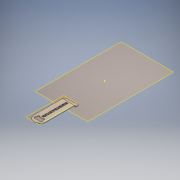
# Autodesk Inventor part: Rost_Heber
Saved by Autodesk Inventor 2018 (Build 220112000, 112)
## iProperties
Created: 2017-10-08
Part Number: Rost_Heber
Material: Generisch
Document SubType Name: Blech
Designer: Jan
Density: 1 g/cm^3
Sheet Metal Rule: Standard_mm
Appearance: Vorgabe
Flat Pattern Width: 4 cm
Flat Pattern Length: 13.3098 cm
Flat Pattern Area: 53.2391 cm^2
Sheet Metal Width: 40,000 mm
Sheet Metal Length: 133,098 mm
Sheet Metal Area: 5323,911 mm^2
Author: Jan
Autodesk Inventor part; units mm, degrees
ref_plane "YZ Plane" through (0, 0, 0) normal (1, 0, 0) x (0, 1, 0)
ref_plane "XZ Plane" through (0, 0, 0) normal (0, 1, 0) x (-1, 0, 0)
ref_plane "XY Plane" through (0, 0, 0) normal (0, 0, 1) x (1, 0, 0)
ref_plane "Arbeitsebene1" through (0, 0, 0) normal (0, 0, 1) x (1, 0, 0)
sketch "Skizze1" plane through (0, 0, 0) normal (0, 0, 1) x (1, 0, 0)
  arc A0 (31.5, -113.5) -> (26.5, -108.5) centre (26.5, -113.5) ccw
  line L0 (26.5, -108.5) -> (-26.5, -108.5)
  arc A1 (-26.5, -108.5) -> (-31.5, -113.5) centre (-26.5, -113.5) ccw
  line L1 (-31.5, -113.5) -> (-31.5, -124.5)
  line L2 (-31.5, -124.5) -> (-71, -124.5)
  arc A2 (-73, -122.5) -> (-71, -124.5) centre (-71, -122.5) ccw
  line L3 (-73, -122.5) -> (-73, 122.5)
  arc A3 (-71, 124.5) -> (-73, 122.5) centre (-71, 122.5) ccw
  line L4 (-71, 124.5) -> (71, 124.5)
  arc A4 (73, 122.5) -> (71, 124.5) centre (71, 122.5) ccw
  line L5 (73, 122.5) -> (73, -122.5)
  arc A5 (71, -124.5) -> (73, -122.5) centre (71, -122.5) ccw
  line L6 (71, -124.5) -> (31.5, -124.5)
  line L7 (31.5, -124.5) -> (31.5, -113.5)
  line L8 (-22.5, -122.5) -> (-22.5, -117.5)
  line L9 (-22.5, -117.5) -> (22.5, -117.5)
  line L10 (22.5, -117.5) -> (22.5, -122.5)
  line L11 (22.5, -122.5) -> (-22.5, -122.5)
  arc A6 (-81, -122.5) -> (-71, -132.5) centre (-71, -122.5) ccw
  line L12 (71, -132.5) -> (-71, -132.5)
  arc A7 (71, -132.5) -> (81, -122.5) centre (71, -122.5) ccw
  line L13 (81, 122.5) -> (81, -122.5)
  arc A8 (81, 122.5) -> (71, 132.5) centre (71, 122.5) ccw
  line L14 (-71, 132.5) -> (71, 132.5)
  arc A9 (-71, 132.5) -> (-81, 122.5) centre (-71, 122.5) ccw
  line L15 (-81, -122.5) -> (-81, 122.5)
  line L16 (-20, -118.5) -> (20, -118.5)
  line L17 (20, -118.5) -> (20, -218.5)
  line L18 (0, -238.5) -> (0, -238.5)
  line L19 (-20, -218.5) -> (-20, -118.5)
  line L20 (-116.2995, 0) -> (116.2995, 0)
  line L21 (0, -314.1009) -> (0, 209.3497)
  arc A10 (-20, -218.5) -> (0, -238.5) centre (0, -218.5) ccw
  arc A11 (0, -238.5) -> (20, -218.5) centre (0, -218.5) ccw
  point P0 (0, 0)
  dimension "HeberBreite" = 40
  dimension "d3" = 1
  dimension "HeberLänge" = 120
  dimension "d5" = 20
  measures "HeberBreite" distance of L16.start L16.end
  measures "d3" distance between parallel lines of L9 L16
  measures "HeberLänge" distance between parallel lines of L18 L16
  measures "d5" radius of A10
extrude "Grobblech1" add sketch "Skizze1" along normal blind 2 contours L21 L11 L19 L16 | L16 L17 L11 L21 | L21 L12 L19 L11 | L11 L17 L12 L21 | L21 A10 L19 L12 | L12 L17 A11 L21
sketch "Skizze2" plane through (20, -120.5, 2) normal (0, 1, 0) x (-1, 0, 0)
  line L0 (40, 0) -> (0, 0)
  line L1 (0, 0) -> (0, -8.05)
  line L2 (0, -8.05) -> (40, -8.05)
  line L3 (40, -8.05) -> (40, 0)
  constraints: 6 end point, 1 horizontal, 1 perpendicular, 1 vertical
edge flange "Lasche1" height 8.05 angle 90 thickness 2 bend radius 2 thickness toward (0, 1, 0) relief straight relief width 2 relief depth 1 edges at (0, -118.5, 0) wall of the first edge with corners at (-20, -120.5, 2) (20, -120.5, 2) (20, -120.5, -6.05) (-20, -120.5, -6.05)
bend "Biegung1"
corner "Ecke1"
sketch "Skizze3" plane through (-20, -120.5, -4.05) normal (0, 0, -1) x (-1, 0, 0)
  line L0 (-40, 0) -> (0, 0)
  line L1 (0, 0) -> (0, 12)
  line L2 (0, 12) -> (-40, 12)
  line L3 (-40, 12) -> (-40, 0)
  constraints: 6 end point, 1 horizontal, 1 perpendicular, 1 vertical
edge flange "Lasche2" height 12 angle 90 thickness 2 bend radius 2 thickness toward (0, 0, -1) relief straight relief width 2 relief depth 1 edges at (0, -118.5, -6.05) wall of the first edge with corners at (20, -120.5, -4.05) (-20, -120.5, -4.05) (-20, -108.5, -4.05) (20, -108.5, -4.05)
bend "Biegung2"
corner "Ecke2"
sketch "Skizze5" plane through (0, 0, 2) normal (0, 0, 1) x (1, 0, 0)
  line L0 (6.947, -214.5463) -> (6.947, -212.4824)
  arc A0 (10.3384, -213.2197) -> (6.947, -212.4824) centre (8.3903, -214.0121) ccw
  line L1 (10.3384, -213.2197) -> (13.6109, -223.4321)
  arc A1 (4.1757, -228.0984) -> (13.6109, -223.4321) centre (7.6304, -223.2116) ccw
  line L2 (20, -122.5) -> (-20, -122.5) projected
  line L3 (-20, -218.5) -> (-20, -122.5) projected
  arc A2 (-20, -218.5) -> (20, -218.5) centre (0, -218.5) ccw projected
  line L4 (20, -122.5) -> (20, -218.5) projected
  line L5 (6.947, -214.5463) -> (-0.053, -214.5463)
  line L6 (4.1757, -228.0984) -> (-0.053, -228.0984)
  arc A3 (-7.053, -212.4824) -> (-10.3568, -213.0318) centre (-8.4962, -214.0121) ccw
  line L7 (-10.3568, -213.0318) -> (-13.7136, -223.5071)
  arc A4 (-13.7136, -223.5071) -> (-4.2816, -228.0984) centre (-7.7363, -223.2116) ccw
  line L8 (-7.053, -214.5463) -> (-0.053, -214.5463)
  line L9 (-4.2816, -228.0984) -> (-0.053, -228.0984)
  line L10 (-7.053, -212.4824) -> (-7.053, -214.5463)
  line L11 (0, -312.7) -> (0, 206.7)
  constraints: 19 end point, 8 point on circle, 4 centre point, 3 parallel, 2 equal radius, 1 point on line, 1 vertical, 2 other
extrude "Ausklinkung1" cut sketch "Skizze5" against normal blind 2 contours L0 A0 L1 A1 L6 L11 L5 | L11 L6 L9 A4 L7 A3 L10 L8 L5
sketch "Skizze7" plane through (0, 0, 2) normal (0, 0, 1) x (1, 0, 0)
  point P0 (0, 0)
ref_plane "Arbeitsebene2" through (0, 0, 7) normal (0, 0, 1) x (1, 0, 0)
sketch "Skizze8" plane through (0, 0, 7) normal (0, 0, 1) x (1, 0, 0)
  line L0 (3.8058, -125.538) -> (3.8058, -288.8575) construction
  line L1 (3.8058, -288.8575) -> (-4.5136, -288.8575) construction
  line L2 (-4.5136, -288.8575) -> (-4.5136, -125.538) construction
  line L3 (-4.5136, -125.538) -> (3.8058, -125.538) construction
  line L4 (3.6661, -129.3965) -> (-3.3339, -129.3965)
  line L5 (-3.3339, -129.3965) -> (-3.3339, -126.6622)
  line L6 (-3.3339, -126.6622) -> (-3.3339, -126.5042)
  spline S0 degree 2 poles (-3.3339, -126.5042) (-3.3339, -126.2794) (-3.1942, -126.0424) (-3.0666, -126.0424) knots 0 0 0 1 2 2 2
  spline S1 degree 2 poles (-3.0666, -126.0424) (-2.86, -126.0424) (-2.7931, -126.2854) knots 0 0 0 1 1 1
  spline S2 degree 2 poles (-2.7931, -126.2854) (-2.7324, -126.492) (-2.7081, -126.5589) (-2.6595, -126.5953) knots 0 0 0 1 2 2 2
  spline S3 degree 2 poles (-2.6595, -126.5953) (-2.5805, -126.6682) (-2.3982, -126.6682) knots 0 0 0 1 1 1
  line L7 (-2.3982, -126.6682) -> (2.7303, -126.6682)
  spline S4 degree 2 poles (2.7303, -126.6682) (2.9126, -126.6682) (2.9916, -126.5953) knots 0 0 0 1 1 1
  spline S5 degree 2 poles (2.9916, -126.5953) (3.0402, -126.5589) (3.0645, -126.492) (3.1192, -126.2854) knots 0 0 0 1 2 2 2
  spline S6 degree 2 poles (3.1192, -126.2854) (3.186, -126.0424) (3.3987, -126.0424) knots 0 0 0 1 1 1
  spline S7 degree 2 poles (3.3987, -126.0424) (3.5263, -126.0424) (3.6661, -126.2794) (3.6661, -126.5042) knots 0 0 0 1 2 2 2
  line L8 (3.6661, -126.5042) -> (3.6661, -126.6622)
  line L9 (3.6661, -126.6622) -> (3.6661, -129.3965)
  line L10 (-3.3339, -129.9556) -> (-2.781, -129.9556)
  spline S8 degree 2 poles (-2.781, -129.9556) (-2.7324, -130.3566) (-2.544, -130.8792) (-2.3556, -131.1405) knots 0 0 0 1 2 2 2
  spline S9 degree 2 poles (-2.3556, -131.1405) (-2.1673, -131.4078) (-1.7602, -131.7177) (-1.4259, -131.8636) knots 0 0 0 1 2 2 2
  spline S10 degree 2 poles (-1.4259, -131.8636) (-1.2619, -131.9304) (-1.1464, -132.0762) (-1.1464, -132.2038) knots 0 0 0 1 2 2 2
  spline S11 degree 2 poles (-1.1464, -132.2038) (-1.1464, -132.3801) (-1.3166, -132.5137) (-1.5232, -132.5137) knots 0 0 0 1 2 2 2
  line L11 (-1.5232, -132.5137) -> (-3.3339, -132.5137)
  line L12 (-3.3339, -132.5137) -> (-3.3339, -129.9556)
  line L13 (3.6661, -129.9495) -> (3.6661, -132.4287)
  line L14 (3.6661, -132.4287) -> (1.8492, -132.4287)
  spline S12 degree 2 poles (1.8492, -132.4287) (1.6912, -132.4287) (1.5515, -132.2828) (1.5515, -132.1188) knots 0 0 0 1 2 2 2
  spline S13 degree 2 poles (1.5515, -132.1188) (1.5515, -131.9851) (1.6426, -131.8636) (1.7885, -131.8089) knots 0 0 0 1 2 2 2
  spline S14 degree 2 poles (1.7885, -131.8089) (2.3779, -131.5719) (3.0037, -130.6665) (3.0645, -129.9495) knots 0 0 0 1 2 2 2
  line L15 (3.0645, -129.9495) -> (3.6661, -129.9495)
  line L16 (-0.0709, -129.9191) -> (0.5246, -129.9191)
  spline S15 degree 2 poles (0.5246, -129.9191) (0.6704, -130.2776) (1.0107, -130.6179) (1.2902, -130.703) knots 0 0 0 1 2 2 2
  spline S16 degree 2 poles (1.2902, -130.703) (1.4846, -130.7516) (1.6366, -130.9096) (1.6366, -131.0554) knots 0 0 0 1 2 2 2
  spline S17 degree 2 poles (1.6366, -131.0554) (1.6366, -131.2559) (1.5089, -131.3288) knots 0 0 0 1 1 1
  spline S18 degree 2 poles (1.5089, -131.3288) (1.4421, -131.3714) (1.2051, -131.3714) knots 0 0 0 1 1 1
  line L17 (1.2051, -131.3714) -> (-0.7515, -131.3714)
  spline S19 degree 2 poles (-0.7515, -131.3714) (-0.9945, -131.3714) (-1.1768, -131.2438) (-1.1768, -131.0676) knots 0 0 0 1 2 2 2
  spline S20 degree 2 poles (-1.1768, -131.0676) (-1.1768, -130.9278) (-1.031, -130.7698) (-0.8608, -130.7212) knots 0 0 0 1 2 2 2
  spline S21 degree 2 poles (-0.8608, -130.7212) (-0.5084, -130.6118) (-0.1317, -130.229) (-0.0709, -129.9191) knots 0 0 0 1 2 2 2
  line L18 (-3.3339, -136.7976) -> (-3.3339, -134.0571)
  line L19 (-3.3339, -134.0571) -> (-3.3339, -133.8992)
  spline S22 degree 2 poles (-3.3339, -133.8992) (-3.3339, -133.6743) (-3.1942, -133.4373) (-3.0666, -133.4373) knots 0 0 0 1 2 2 2
  spline S23 degree 2 poles (-3.0666, -133.4373) (-2.86, -133.4373) (-2.7931, -133.6804) knots 0 0 0 1 1 1
  spline S24 degree 2 poles (-2.7931, -133.6804) (-2.7324, -133.887) (-2.7081, -133.9538) (-2.6595, -133.9903) knots 0 0 0 1 2 2 2
  spline S25 degree 2 poles (-2.6595, -133.9903) (-2.5805, -134.0632) (-2.3982, -134.0632) knots 0 0 0 1 1 1
  line L20 (-2.3982, -134.0632) -> (2.7303, -134.0632)
  spline S26 degree 2 poles (2.7303, -134.0632) (2.9126, -134.0632) (2.9916, -133.9903) knots 0 0 0 1 1 1
  spline S27 degree 2 poles (2.9916, -133.9903) (3.0402, -133.9538) (3.0645, -133.887) (3.1192, -133.6804) knots 0 0 0 1 2 2 2
  spline S28 degree 2 poles (3.1192, -133.6804) (3.186, -133.4373) (3.3987, -133.4373) knots 0 0 0 1 1 1
  spline S29 degree 2 poles (3.3987, -133.4373) (3.5263, -133.4373) (3.6661, -133.6743) (3.6661, -133.8992) knots 0 0 0 1 2 2 2
  line L21 (3.6661, -133.8992) -> (3.6661, -134.0571)
  line L22 (3.6661, -134.0571) -> (3.6661, -136.7976)
  line L23 (3.6661, -136.7976) -> (3.6661, -136.9556)
  spline S30 degree 2 poles (3.6661, -136.9556) (3.6661, -137.1804) (3.5263, -137.4174) (3.3987, -137.4174) knots 0 0 0 1 2 2 2
  spline S31 degree 2 poles (3.3987, -137.4174) (3.186, -137.4174) (3.1192, -137.1743) knots 0 0 0 1 1 1
  spline S32 degree 2 poles (3.1192, -137.1743) (3.0645, -136.9677) (3.0402, -136.9009) (2.9916, -136.8644) knots 0 0 0 1 2 2 2
  spline S33 degree 2 poles (2.9916, -136.8644) (2.9126, -136.7915) (2.7303, -136.7915) knots 0 0 0 1 1 1
  line L24 (2.7303, -136.7915) -> (-2.3982, -136.7915)
  spline S34 degree 2 poles (-2.3982, -136.7915) (-2.5805, -136.7915) (-2.6595, -136.8644) knots 0 0 0 1 1 1
  spline S35 degree 2 poles (-2.6595, -136.8644) (-2.7081, -136.9009) (-2.7324, -136.9677) (-2.7931, -137.1743) knots 0 0 0 1 2 2 2
  spline S36 degree 2 poles (-2.7931, -137.1743) (-2.86, -137.4174) (-3.0666, -137.4174) knots 0 0 0 1 1 1
  spline S37 degree 2 poles (-3.0666, -137.4174) (-3.1942, -137.4174) (-3.3339, -137.1804) (-3.3339, -136.9556) knots 0 0 0 1 2 2 2
  line L25 (-3.3339, -136.9556) -> (-3.3339, -136.7976)
  line L26 (3.8058, -141.2698) -> (3.2164, -141.2698)
  spline S38 degree 2 poles (3.2164, -141.2698) (3.1253, -140.887) (2.7607, -140.486) (2.4994, -140.486) knots 0 0 0 1 2 2 2
  spline S39 degree 2 poles (2.4994, -140.486) (2.2381, -140.486) (1.8553, -140.8202) (1.6791, -141.1908) knots 0 0 0 1 2 2 2
  spline S40 degree 2 poles (1.6791, -141.1908) (1.5636, -141.4521) (1.2294, -142.3636) knots 0 0 0 1 1 1
  spline S41 degree 2 poles (1.2294, -142.3636) (1.0289, -142.9165) (0.7069, -143.5242) (0.4638, -143.7976) knots 0 0 0 1 2 2 2
  spline S42 degree 2 poles (0.4638, -143.7976) (-0.1681, -144.5207) (-1.0492, -144.5207) knots 0 0 0 1 1 1
  spline S43 degree 2 poles (-1.0492, -144.5207) (-1.7055, -144.5207) (-2.8053, -143.7307) (-3.1213, -143.0441) knots 0 0 0 1 2 2 2
  spline S44 degree 2 poles (-3.1213, -143.0441) (-3.2853, -142.6735) (-3.4737, -141.7985) (-3.4737, -141.4156) knots 0 0 0 1 2 2 2
  line L27 (-3.4737, -141.4156) -> (-2.8904, -141.4156)
  spline S45 degree 2 poles (-2.8904, -141.4156) (-2.781, -141.9504) (-2.3982, -142.4243) (-2.07, -142.4243) knots 0 0 0 1 2 2 2
  spline S46 degree 2 poles (-2.07, -142.4243) (-1.7237, -142.4243) (-1.4624, -142.0537) knots 0 0 0 1 1 1
  spline S47 degree 2 poles (-1.4624, -142.0537) (-1.2923, -141.8106) (-1.0431, -141.1179) knots 0 0 0 1 1 1
  spline S48 degree 2 poles (-1.0431, -141.1179) (-0.7636, -140.3644) (-0.5266, -139.8054) (-0.3687, -139.5441) knots 0 0 0 1 2 2 2
  spline S49 degree 2 poles (-0.3687, -139.5441) (0.318, -138.3896) (1.4603, -138.3896) knots 0 0 0 1 1 1
  spline S50 degree 2 poles (1.4603, -138.3896) (2.0437, -138.3896) (3.0341, -138.9669) (3.3379, -139.4834) knots 0 0 0 1 2 2 2
  spline S51 degree 2 poles (3.3379, -139.4834) (3.7572, -140.2064) (3.8058, -141.2698) knots 0 0 0 1 1 1
  line L28 (-2.8904, -140.9478) -> (-3.4737, -140.9478)
  spline S52 degree 2 poles (-3.4737, -140.9478) (-3.4737, -140.4434) (-3.2367, -139.8358) knots 0 0 0 1 1 1
  spline S53 degree 2 poles (-3.2367, -139.8358) (-3.1456, -139.6049) (-3.097, -139.4347) (-3.097, -139.3557) knots 0 0 0 1 2 2 2
  spline S54 degree 2 poles (-3.097, -139.3557) (-3.097, -139.2342) (-3.1638, -139.1066) (-3.2975, -138.9729) knots 0 0 0 1 2 2 2
  spline S55 degree 2 poles (-3.2975, -138.9729) (-3.4069, -138.8636) (-3.4069, -138.736) knots 0 0 0 1 1 1
  spline S56 degree 2 poles (-3.4069, -138.736) (-3.4069, -138.3896) (-2.9633, -138.3896) knots 0 0 0 1 1 1
  line L29 (-2.9633, -138.3896) -> (-1.0978, -138.3896)
  spline S57 degree 2 poles (-1.0978, -138.3896) (-0.9581, -138.3896) (-0.7575, -138.584) (-0.7515, -138.736) knots 0 0 0 1 2 2 2
  spline S58 degree 2 poles (-0.7515, -138.736) (-0.7454, -138.8696) (-0.8852, -139.0215) (-1.0614, -139.0762) knots 0 0 0 1 2 2 2
  spline S59 degree 2 poles (-1.0614, -139.0762) (-1.4989, -139.2221) (-2.2706, -139.7568) (-2.5319, -140.1092) knots 0 0 0 1 2 2 2
  spline S60 degree 2 poles (-2.5319, -140.1092) (-2.8114, -140.4738) (-2.8904, -140.9478) knots 0 0 0 1 1 1
  line L30 (3.2164, -141.7559) -> (3.7815, -141.7559)
  spline S61 degree 2 poles (3.7815, -141.7559) (3.7572, -142.1266) (3.6357, -142.6674) (3.4595, -143.1656) knots 0 0 0 1 2 2 2
  spline S62 degree 2 poles (3.4595, -143.1656) (3.4169, -143.2872) (3.4169, -143.3662) knots 0 0 0 1 1 1
  spline S63 degree 2 poles (3.4169, -143.3662) (3.4169, -143.4816) (3.4838, -143.5424) knots 0 0 0 1 1 1
  line L31 (3.4838, -143.5424) -> (3.6357, -143.6761)
  spline S64 degree 2 poles (3.6357, -143.6761) (3.7511, -143.7733) (3.7511, -143.913) knots 0 0 0 1 1 1
  spline S65 degree 2 poles (3.7511, -143.913) (3.7511, -144.0832) (3.5506, -144.2351) (3.3379, -144.2351) knots 0 0 0 1 2 2 2
  line L32 (3.3379, -144.2351) -> (1.6426, -144.2351)
  spline S66 degree 2 poles (1.6426, -144.2351) (1.4907, -144.2351) (1.3023, -144.0346) (1.3023, -143.8705) knots 0 0 0 1 2 2 2
  spline S67 degree 2 poles (1.3023, -143.8705) (1.3023, -143.749) (1.3692, -143.6457) knots 0 0 0 1 1 1
  spline S68 degree 2 poles (1.3692, -143.6457) (1.4117, -143.591) (1.5272, -143.5242) (1.6669, -143.4938) knots 0 0 0 1 2 2 2
  spline S69 degree 2 poles (1.6669, -143.4938) (1.9221, -143.4209) (2.4508, -143.0927) (2.6635, -142.8679) knots 0 0 0 1 2 2 2
  spline S70 degree 2 poles (2.6635, -142.8679) (3.0827, -142.4243) (3.2164, -141.7559) knots 0 0 0 1 1 1
  line L33 (3.6661, -148.841) -> (-3.3339, -148.841)
  line L34 (-3.3339, -148.841) -> (-3.3339, -146.1066)
  line L35 (-3.3339, -146.1066) -> (-3.3339, -145.9486)
  spline S71 degree 2 poles (-3.3339, -145.9486) (-3.3339, -145.7238) (-3.1942, -145.4868) (-3.0666, -145.4868) knots 0 0 0 1 2 2 2
  spline S72 degree 2 poles (-3.0666, -145.4868) (-2.86, -145.4868) (-2.7931, -145.7299) knots 0 0 0 1 1 1
  spline S73 degree 2 poles (-2.7931, -145.7299) (-2.7324, -145.9365) (-2.7081, -146.0033) (-2.6595, -146.0398) knots 0 0 0 1 2 2 2
  spline S74 degree 2 poles (-2.6595, -146.0398) (-2.5805, -146.1127) (-2.3982, -146.1127) knots 0 0 0 1 1 1
  line L36 (-2.3982, -146.1127) -> (2.7303, -146.1127)
  spline S75 degree 2 poles (2.7303, -146.1127) (2.9126, -146.1127) (2.9916, -146.0398) knots 0 0 0 1 1 1
  spline S76 degree 2 poles (2.9916, -146.0398) (3.0402, -146.0033) (3.0645, -145.9365) (3.1192, -145.7299) knots 0 0 0 1 2 2 2
  spline S77 degree 2 poles (3.1192, -145.7299) (3.186, -145.4868) (3.3987, -145.4868) knots 0 0 0 1 1 1
  spline S78 degree 2 poles (3.3987, -145.4868) (3.5263, -145.4868) (3.6661, -145.7238) (3.6661, -145.9486) knots 0 0 0 1 2 2 2
  line L37 (3.6661, -145.9486) -> (3.6661, -146.1066)
  line L38 (3.6661, -146.1066) -> (3.6661, -148.841)
  line L39 (-3.3339, -149.4) -> (-2.781, -149.4)
  spline S79 degree 2 poles (-2.781, -149.4) (-2.7324, -149.8011) (-2.544, -150.3236) (-2.3556, -150.5849) knots 0 0 0 1 2 2 2
  spline S80 degree 2 poles (-2.3556, -150.5849) (-2.1673, -150.8523) (-1.7602, -151.1622) (-1.4259, -151.308) knots 0 0 0 1 2 2 2
  spline S81 degree 2 poles (-1.4259, -151.308) (-1.2619, -151.3748) (-1.1464, -151.5207) (-1.1464, -151.6483) knots 0 0 0 1 2 2 2
  spline S82 degree 2 poles (-1.1464, -151.6483) (-1.1464, -151.8245) (-1.3166, -151.9582) (-1.5232, -151.9582) knots 0 0 0 1 2 2 2
  line L40 (-1.5232, -151.9582) -> (-3.3339, -151.9582)
  line L41 (-3.3339, -151.9582) -> (-3.3339, -149.4)
  line L42 (3.6661, -149.3939) -> (3.6661, -151.8731)
  line L43 (3.6661, -151.8731) -> (1.8492, -151.8731)
  spline S83 degree 2 poles (1.8492, -151.8731) (1.6912, -151.8731) (1.5515, -151.7273) (1.5515, -151.5632) knots 0 0 0 1 2 2 2
  spline S84 degree 2 poles (1.5515, -151.5632) (1.5515, -151.4295) (1.6426, -151.308) (1.7885, -151.2533) knots 0 0 0 1 2 2 2
  spline S85 degree 2 poles (1.7885, -151.2533) (2.3779, -151.0163) (3.0037, -150.111) (3.0645, -149.3939) knots 0 0 0 1 2 2 2
  line L44 (3.0645, -149.3939) -> (3.6661, -149.3939)
  line L45 (-0.0709, -149.3636) -> (0.5246, -149.3636)
  spline S86 degree 2 poles (0.5246, -149.3636) (0.6704, -149.7221) (1.0107, -150.0623) (1.2902, -150.1474) knots 0 0 0 1 2 2 2
  spline S87 degree 2 poles (1.2902, -150.1474) (1.4846, -150.196) (1.6366, -150.354) (1.6366, -150.4998) knots 0 0 0 1 2 2 2
  spline S88 degree 2 poles (1.6366, -150.4998) (1.6366, -150.7004) (1.5089, -150.7733) knots 0 0 0 1 1 1
  spline S89 degree 2 poles (1.5089, -150.7733) (1.4421, -150.8158) (1.2051, -150.8158) knots 0 0 0 1 1 1
  line L46 (1.2051, -150.8158) -> (-0.7515, -150.8158)
  spline S90 degree 2 poles (-0.7515, -150.8158) (-0.9945, -150.8158) (-1.1768, -150.6882) (-1.1768, -150.512) knots 0 0 0 1 2 2 2
  spline S91 degree 2 poles (-1.1768, -150.512) (-1.1768, -150.3722) (-1.031, -150.2143) (-0.8608, -150.1656) knots 0 0 0 1 2 2 2
  spline S92 degree 2 poles (-0.8608, -150.1656) (-0.5084, -150.0563) (-0.1317, -149.6735) (-0.0709, -149.3636) knots 0 0 0 1 2 2 2
  line L47 (3.6661, -156.3636) -> (-1.0735, -159.6327)
  line L48 (-1.0735, -159.6327) -> (-3.3339, -159.6327)
  line L49 (-3.3339, -159.6327) -> (-3.3339, -157.9556)
  line L50 (-3.3339, -157.9556) -> (2.6635, -153.7811)
  spline S93 degree 2 poles (2.6635, -153.7811) (2.864, -153.6413) (3.0159, -153.4712) (3.0523, -153.3375) knots 0 0 0 1 2 2 2
  line L51 (3.0523, -153.3375) -> (3.1253, -153.1005)
  spline S94 degree 2 poles (3.1253, -153.1005) (3.1496, -153.0094) (3.2833, -152.9) (3.3622, -152.9) knots 0 0 0 1 2 2 2
  spline S95 degree 2 poles (3.3622, -152.9) (3.4534, -152.9) (3.5992, -153.0094) (3.6296, -153.1005) knots 0 0 0 1 2 2 2
  spline S96 degree 2 poles (3.6296, -153.1005) (3.6661, -153.2038) (3.6661, -153.6656) knots 0 0 0 1 1 1
  line L52 (3.6661, -153.6656) -> (3.6661, -156.3636)
  line L53 (1.8614, -153.7872) -> (0.9621, -154.4373)
  line L54 (0.9621, -154.4373) -> (-1.7845, -154.4373)
  spline S97 degree 2 poles (-1.7845, -154.4373) (-2.143, -154.4373) (-2.6048, -154.729) (-2.7567, -155.0389) knots 0 0 0 1 2 2 2
  line L55 (-2.7567, -155.0389) -> (-2.8417, -155.2273)
  spline S98 degree 2 poles (-2.8417, -155.2273) (-2.9207, -155.3853) (-3.0727, -155.3853) knots 0 0 0 1 1 1
  spline S99 degree 2 poles (-3.0727, -155.3853) (-3.1881, -155.3853) (-3.2671, -155.2698) knots 0 0 0 1 1 1
  spline S100 degree 2 poles (-3.2671, -155.2698) (-3.3339, -155.1726) (-3.3339, -154.8627) knots 0 0 0 1 1 1
  line L56 (-3.3339, -154.8627) -> (-3.3339, -153.4408)
  spline S101 degree 2 poles (-3.3339, -153.4408) (-3.3339, -152.8818) (-3.0666, -152.8818) knots 0 0 0 1 1 1
  spline S102 degree 2 poles (-3.0666, -152.8818) (-2.9754, -152.8818) (-2.8661, -152.9972) (-2.7749, -153.1978) knots 0 0 0 1 2 2 2
  spline S103 degree 2 poles (-2.7749, -153.1978) (-2.5015, -153.7872) (-1.7845, -153.7872) knots 0 0 0 1 1 1
  line L57 (-1.7845, -153.7872) -> (1.8614, -153.7872)
  line L58 (-0.2532, -159.6327) -> (0.6643, -158.9825)
  line L59 (0.6643, -158.9825) -> (2.0862, -158.9825)
  spline S104 degree 2 poles (2.0862, -158.9825) (2.5176, -158.9825) (2.9734, -158.6787) (3.1374, -158.3019) knots 0 0 0 1 2 2 2
  spline S105 degree 2 poles (3.1374, -158.3019) (3.186, -158.1682) (3.3076, -158.071) (3.3987, -158.071) knots 0 0 0 1 2 2 2
  spline S106 degree 2 poles (3.3987, -158.071) (3.5385, -158.071) (3.6661, -158.2898) (3.6661, -158.5268) knots 0 0 0 1 2 2 2
  line L60 (3.6661, -158.5268) -> (3.6661, -160.0641)
  spline S107 degree 2 poles (3.6661, -160.0641) (3.6661, -160.3801) (3.581, -160.4773) knots 0 0 0 1 1 1
  spline S108 degree 2 poles (3.581, -160.4773) (3.502, -160.5806) (3.3866, -160.5806) knots 0 0 0 1 1 1
  spline S109 degree 2 poles (3.3866, -160.5806) (3.2833, -160.5806) (3.1739, -160.4651) (3.0827, -160.2403) knots 0 0 0 1 2 2 2
  spline S110 degree 2 poles (3.0827, -160.2403) (2.943, -159.9182) (2.6574, -159.7481) knots 0 0 0 1 1 1
  spline S111 degree 2 poles (2.6574, -159.7481) (2.4447, -159.6327) (2.0862, -159.6327) knots 0 0 0 1 1 1
  line L61 (2.0862, -159.6327) -> (-0.2532, -159.6327)
  line L62 (3.6661, -164.6943) -> (-3.3339, -164.6943)
  line L63 (-3.3339, -164.6943) -> (-3.3339, -161.9599)
  line L64 (-3.3339, -161.9599) -> (-3.3339, -161.8019)
  spline S112 degree 2 poles (-3.3339, -161.8019) (-3.3339, -161.5771) (-3.1942, -161.3401) (-3.0666, -161.3401) knots 0 0 0 1 2 2 2
  spline S113 degree 2 poles (-3.0666, -161.3401) (-2.86, -161.3401) (-2.7931, -161.5832) knots 0 0 0 1 1 1
  spline S114 degree 2 poles (-2.7931, -161.5832) (-2.7324, -161.7898) (-2.7081, -161.8566) (-2.6595, -161.8931) knots 0 0 0 1 2 2 2
  spline S115 degree 2 poles (-2.6595, -161.8931) (-2.5805, -161.966) (-2.3982, -161.966) knots 0 0 0 1 1 1
  line L65 (-2.3982, -161.966) -> (2.7303, -161.966)
  spline S116 degree 2 poles (2.7303, -161.966) (2.9126, -161.966) (2.9916, -161.8931) knots 0 0 0 1 1 1
  spline S117 degree 2 poles (2.9916, -161.8931) (3.0402, -161.8566) (3.0645, -161.7898) (3.1192, -161.5832) knots 0 0 0 1 2 2 2
  spline S118 degree 2 poles (3.1192, -161.5832) (3.186, -161.3401) (3.3987, -161.3401) knots 0 0 0 1 1 1
  spline S119 degree 2 poles (3.3987, -161.3401) (3.5263, -161.3401) (3.6661, -161.5771) (3.6661, -161.8019) knots 0 0 0 1 2 2 2
  line L66 (3.6661, -161.8019) -> (3.6661, -161.9599)
  line L67 (3.6661, -161.9599) -> (3.6661, -164.6943)
  spline S120 degree 2 poles (0.2876, -166.6084) (0.1964, -167.1613) (0.0263, -167.7629) (-0.1074, -167.9998) knots 0 0 0 1 2 2 2
  spline S121 degree 2 poles (-0.1074, -167.9998) (-0.3322, -168.413) (-1.0553, -168.8505) (-1.4989, -168.8505) knots 0 0 0 1 2 2 2
  spline S122 degree 2 poles (-1.4989, -168.8505) (-2.3739, -168.8505) (-2.8661, -168.0728) knots 0 0 0 1 1 1
  spline S123 degree 2 poles (-2.8661, -168.0728) (-3.1213, -167.6778) (-3.3339, -166.7116) (-3.3339, -165.9278) knots 0 0 0 1 2 2 2
  line L68 (-3.3339, -165.9278) -> (-3.3339, -165.1926)
  line L69 (-3.3339, -165.1926) -> (-2.7931, -165.1926)
  spline S124 degree 2 poles (-2.7931, -165.1926) (-2.781, -165.4417) (-2.6959, -165.7212) (-2.5926, -165.8366) knots 0 0 0 1 2 2 2
  spline S125 degree 2 poles (-2.5926, -165.8366) (-2.3982, -166.0372) (-2.0032, -166.0372) knots 0 0 0 1 1 1
  line L70 (-2.0032, -166.0372) -> (-0.8365, -166.0372)
  spline S126 degree 2 poles (-0.8365, -166.0372) (-0.5813, -166.0372) (-0.2957, -165.9339) (-0.1742, -165.7941) knots 0 0 0 1 2 2 2
  spline S127 degree 2 poles (-0.1742, -165.7941) (-0.0831, -165.6908) (-0.0041, -165.4417) (0.0263, -165.2169) knots 0 0 0 1 2 2 2
  line L71 (0.0263, -165.2169) -> (0.555, -165.2169)
  spline S128 degree 2 poles (0.555, -165.2169) (0.5732, -165.4417) (0.6461, -165.6969) (0.7251, -165.8002) knots 0 0 0 1 2 2 2
  spline S129 degree 2 poles (0.7251, -165.8002) (0.8041, -165.8974) (1.0471, -166.0311) (1.1504, -166.0372) knots 0 0 0 1 2 2 2
  line L72 (1.1504, -166.0372) -> (1.436, -166.0372)
  line L73 (1.436, -166.0372) -> (2.3232, -166.0372)
  spline S130 degree 2 poles (2.3232, -166.0372) (2.4629, -166.0372) (2.7668, -165.9278) (2.8518, -165.8488) knots 0 0 0 1 2 2 2
  spline S131 degree 2 poles (2.8518, -165.8488) (2.9673, -165.7273) (3.0827, -165.4417) (3.101, -165.1926) knots 0 0 0 1 2 2 2
  line L74 (3.101, -165.1926) -> (3.6661, -165.1926)
  line L75 (3.6661, -165.1926) -> (3.6661, -165.9035)
  spline S132 degree 2 poles (3.6661, -165.9035) (3.6661, -167.3071) (3.186, -168.0424) knots 0 0 0 1 1 1
  spline S133 degree 2 poles (3.186, -168.0424) (2.9612, -168.3827) (2.3353, -168.7412) (1.9708, -168.7412) knots 0 0 0 1 2 2 2
  spline S134 degree 2 poles (1.9708, -168.7412) (1.6122, -168.7412) (0.9803, -168.3766) (0.7676, -168.0485) knots 0 0 0 1 2 2 2
  spline S135 degree 2 poles (0.7676, -168.0485) (0.6036, -167.8115) (0.397, -167.1856) (0.2876, -166.6084) knots 0 0 0 1 2 2 2
  line L76 (3.6661, -172.2412) -> (3.6661, -174.7203)
  line L77 (3.6661, -174.7203) -> (-2.3617, -176.4278)
  spline S136 degree 2 poles (-2.3617, -176.4278) (-2.5197, -176.4764) (-2.6412, -176.5372) knots 0 0 0 1 1 1
  spline S137 degree 2 poles (-2.6412, -176.5372) (-2.7384, -176.5919) (-2.7992, -176.7863) knots 0 0 0 1 1 1
  spline S138 degree 2 poles (-2.7992, -176.7863) (-2.86, -176.9443) (-2.9694, -177.0658) (-3.0666, -177.0658) knots 0 0 0 1 2 2 2
  spline S139 degree 2 poles (-3.0666, -177.0658) (-3.3339, -177.0658) (-3.3339, -176.5919) knots 0 0 0 1 1 1
  line L78 (-3.3339, -176.5919) -> (-3.3339, -173.5172)
  spline S140 degree 2 poles (-3.3339, -173.5172) (-3.3339, -173.3349) (-3.182, -173.1162) (-3.0605, -173.1162) knots 0 0 0 1 2 2 2
  spline S141 degree 2 poles (-3.0605, -173.1162) (-2.9572, -173.1162) (-2.8539, -173.2134) (-2.781, -173.3896) knots 0 0 0 1 2 2 2
  spline S142 degree 2 poles (-2.781, -173.3896) (-2.7263, -173.5111) (-2.6048, -173.6084) (-2.5136, -173.6084) knots 0 0 0 1 2 2 2
  spline S143 degree 2 poles (-2.5136, -173.6084) (-2.4225, -173.6084) (-2.3556, -173.5901) knots 0 0 0 1 1 1
  line L79 (-2.3556, -173.5901) -> (-1.6143, -173.3896)
  line L80 (-1.6143, -173.3896) -> (-1.6143, -171.6761)
  line L81 (-1.6143, -171.6761) -> (-1.0067, -171.8401)
  line L82 (-1.0067, -171.8401) -> (-1.0067, -173.2195)
  line L83 (-1.0067, -173.2195) -> (3.1617, -172.0893)
  line L84 (3.1617, -172.0893) -> (3.6661, -172.2412)
  line L85 (2.3596, -171.8158) -> (1.3023, -172.1318)
  line L86 (1.3023, -172.1318) -> (-2.0093, -171.038)
  spline S144 degree 2 poles (-2.0093, -171.038) (-2.1551, -170.9894) (-2.2766, -170.9894) knots 0 0 0 1 1 1
  spline S145 degree 2 poles (-2.2766, -170.9894) (-2.5987, -170.9894) (-2.7384, -171.354) knots 0 0 0 1 1 1
  line L87 (-2.7384, -171.354) -> (-2.8235, -171.5667)
  spline S146 degree 2 poles (-2.8235, -171.5667) (-2.8964, -171.7733) (-3.0787, -171.7733) knots 0 0 0 1 1 1
  spline S147 degree 2 poles (-3.0787, -171.7733) (-3.3339, -171.7733) (-3.3339, -171.3236) knots 0 0 0 1 1 1
  line L88 (-3.3339, -171.3236) -> (-3.3339, -169.762)
  spline S148 degree 2 poles (-3.3339, -169.762) (-3.3339, -169.5372) (-3.1759, -169.2698) (-3.0362, -169.2698) knots 0 0 0 1 2 2 2
  spline S149 degree 2 poles (-3.0362, -169.2698) (-2.8904, -169.2698) (-2.7931, -169.5432) knots 0 0 0 1 1 1
  spline S150 degree 2 poles (-2.7931, -169.5432) (-2.6959, -169.7924) (-2.5501, -170.0354) (-2.4225, -170.1448) knots 0 0 0 1 2 2 2
  spline S151 degree 2 poles (-2.4225, -170.1448) (-2.2098, -170.3149) (-1.8634, -170.4243) knots 0 0 0 1 1 1
  line L89 (-1.8634, -170.4243) -> (2.3596, -171.8158)
  line L90 (0.4942, -181.5866) -> (0.4942, -182.5893)
  line L91 (0.4942, -182.5893) -> (2.7303, -182.5893)
  spline S152 degree 2 poles (2.7303, -182.5893) (3.022, -182.5893) (3.0706, -182.413) knots 0 0 0 1 1 1
  line L92 (3.0706, -182.413) -> (3.1192, -182.2125)
  spline S153 degree 2 poles (3.1192, -182.2125) (3.186, -181.9816) (3.3987, -181.9816) knots 0 0 0 1 1 1
  spline S154 degree 2 poles (3.3987, -181.9816) (3.6661, -181.9816) (3.6661, -182.4252) knots 0 0 0 1 1 1
  line L93 (3.6661, -182.4252) -> (3.6661, -182.5832)
  line L94 (3.6661, -182.5832) -> (3.6661, -185.3176)
  line L95 (3.6661, -185.3176) -> (3.6661, -185.4816)
  spline S155 degree 2 poles (3.6661, -185.4816) (3.6661, -185.9434) (3.3987, -185.9434) knots 0 0 0 1 1 1
  spline S156 degree 2 poles (3.3987, -185.9434) (3.186, -185.9434) (3.1192, -185.7004) knots 0 0 0 1 1 1
  spline S157 degree 2 poles (3.1192, -185.7004) (3.0645, -185.4938) (3.0402, -185.4269) (2.9916, -185.3905) knots 0 0 0 1 2 2 2
  spline S158 degree 2 poles (2.9916, -185.3905) (2.9126, -185.3176) (2.7303, -185.3176) knots 0 0 0 1 1 1
  line L96 (2.7303, -185.3176) -> (-2.3799, -185.3176)
  spline S159 degree 2 poles (-2.3799, -185.3176) (-2.6655, -185.3176) (-2.7263, -185.4998) knots 0 0 0 1 1 1
  line L97 (-2.7263, -185.4998) -> (-2.781, -185.7004)
  spline S160 degree 2 poles (-2.781, -185.7004) (-2.8478, -185.9434) (-3.0605, -185.9434) knots 0 0 0 1 1 1
  spline S161 degree 2 poles (-3.0605, -185.9434) (-3.3339, -185.9434) (-3.3339, -185.4816) knots 0 0 0 1 1 1
  line L98 (-3.3339, -185.4816) -> (-3.3339, -185.3176)
  line L99 (-3.3339, -185.3176) -> (-3.3339, -182.5832)
  line L100 (-3.3339, -182.5832) -> (-3.3339, -182.413)
  spline S162 degree 2 poles (-3.3339, -182.413) (-3.3339, -181.9816) (-3.0605, -181.9816) knots 0 0 0 1 1 1
  spline S163 degree 2 poles (-3.0605, -181.9816) (-2.8478, -181.9816) (-2.781, -182.2125) knots 0 0 0 1 1 1
  line L101 (-2.781, -182.2125) -> (-2.7263, -182.413)
  spline S164 degree 2 poles (-2.7263, -182.413) (-2.6777, -182.5893) (-2.3799, -182.5893) knots 0 0 0 1 1 1
  line L102 (-2.3799, -182.5893) -> (-0.0162, -182.5893)
  line L103 (-0.0162, -182.5893) -> (-0.0162, -181.5866)
  line L104 (-0.0162, -181.5866) -> (0.4942, -181.5866)
  line L105 (-3.3339, -181.0702) -> (-3.3339, -178.3297)
  line L106 (-3.3339, -178.3297) -> (-3.3339, -178.1717)
  spline S165 degree 2 poles (-3.3339, -178.1717) (-3.3339, -177.9469) (-3.1942, -177.7099) (-3.0666, -177.7099) knots 0 0 0 1 2 2 2
  spline S166 degree 2 poles (-3.0666, -177.7099) (-2.86, -177.7099) (-2.7931, -177.953) knots 0 0 0 1 1 1
  spline S167 degree 2 poles (-2.7931, -177.953) (-2.7324, -178.1596) (-2.7081, -178.2264) (-2.6595, -178.2629) knots 0 0 0 1 2 2 2
  spline S168 degree 2 poles (-2.6595, -178.2629) (-2.5805, -178.3358) (-2.3982, -178.3358) knots 0 0 0 1 1 1
  line L107 (-2.3982, -178.3358) -> (2.7303, -178.3358)
  spline S169 degree 2 poles (2.7303, -178.3358) (2.9126, -178.3358) (2.9916, -178.2629) knots 0 0 0 1 1 1
  spline S170 degree 2 poles (2.9916, -178.2629) (3.0402, -178.2264) (3.0645, -178.1596) (3.1192, -177.953) knots 0 0 0 1 2 2 2
  spline S171 degree 2 poles (3.1192, -177.953) (3.186, -177.7099) (3.3987, -177.7099) knots 0 0 0 1 1 1
  spline S172 degree 2 poles (3.3987, -177.7099) (3.5263, -177.7099) (3.6661, -177.9469) (3.6661, -178.1717) knots 0 0 0 1 2 2 2
  line L108 (3.6661, -178.1717) -> (3.6661, -178.3297)
  line L109 (3.6661, -178.3297) -> (3.6661, -181.0702)
  line L110 (3.6661, -181.0702) -> (3.6661, -181.2281)
  spline S173 degree 2 poles (3.6661, -181.2281) (3.6661, -181.6656) (3.3987, -181.6656) knots 0 0 0 1 1 1
  spline S174 degree 2 poles (3.3987, -181.6656) (3.186, -181.6656) (3.1192, -181.4347) knots 0 0 0 1 1 1
  line L111 (3.1192, -181.4347) -> (3.0706, -181.2403)
  spline S175 degree 2 poles (3.0706, -181.2403) (3.022, -181.0641) (2.7303, -181.0641) knots 0 0 0 1 1 1
  line L112 (2.7303, -181.0641) -> (-2.3982, -181.0641)
  spline S176 degree 2 poles (-2.3982, -181.0641) (-2.6898, -181.0641) (-2.7384, -181.2403) knots 0 0 0 1 1 1
  line L113 (-2.7384, -181.2403) -> (-2.7931, -181.4347)
  spline S177 degree 2 poles (-2.7931, -181.4347) (-2.8539, -181.6656) (-3.0666, -181.6656) knots 0 0 0 1 1 1
  spline S178 degree 2 poles (-3.0666, -181.6656) (-3.3339, -181.6656) (-3.3339, -181.2281) knots 0 0 0 1 1 1
  line L114 (-3.3339, -181.2281) -> (-3.3339, -181.0702)
  line L115 (3.6661, -190.5676) -> (-1.0735, -193.8366)
  line L116 (-1.0735, -193.8366) -> (-3.3339, -193.8366)
  line L117 (-3.3339, -193.8366) -> (-3.3339, -192.1596)
  line L118 (-3.3339, -192.1596) -> (2.6635, -187.9851)
  spline S179 degree 2 poles (2.6635, -187.9851) (2.864, -187.8453) (3.0159, -187.6752) (3.0523, -187.5415) knots 0 0 0 1 2 2 2
  line L119 (3.0523, -187.5415) -> (3.1253, -187.3045)
  spline S180 degree 2 poles (3.1253, -187.3045) (3.1496, -187.2134) (3.2833, -187.104) (3.3622, -187.104) knots 0 0 0 1 2 2 2
  spline S181 degree 2 poles (3.3622, -187.104) (3.4534, -187.104) (3.5992, -187.2134) (3.6296, -187.3045) knots 0 0 0 1 2 2 2
  spline S182 degree 2 poles (3.6296, -187.3045) (3.6661, -187.4078) (3.6661, -187.8696) knots 0 0 0 1 1 1
  line L120 (3.6661, -187.8696) -> (3.6661, -190.5676)
  line L121 (1.8614, -187.9912) -> (0.9621, -188.6413)
  line L122 (0.9621, -188.6413) -> (-1.7845, -188.6413)
  spline S183 degree 2 poles (-1.7845, -188.6413) (-2.143, -188.6413) (-2.6048, -188.933) (-2.7567, -189.2429) knots 0 0 0 1 2 2 2
  line L123 (-2.7567, -189.2429) -> (-2.8417, -189.4313)
  spline S184 degree 2 poles (-2.8417, -189.4313) (-2.9207, -189.5893) (-3.0727, -189.5893) knots 0 0 0 1 1 1
  spline S185 degree 2 poles (-3.0727, -189.5893) (-3.1881, -189.5893) (-3.2671, -189.4738) knots 0 0 0 1 1 1
  spline S186 degree 2 poles (-3.2671, -189.4738) (-3.3339, -189.3766) (-3.3339, -189.0667) knots 0 0 0 1 1 1
  line L124 (-3.3339, -189.0667) -> (-3.3339, -187.6448)
  spline S187 degree 2 poles (-3.3339, -187.6448) (-3.3339, -187.0858) (-3.0666, -187.0858) knots 0 0 0 1 1 1
  spline S188 degree 2 poles (-3.0666, -187.0858) (-2.9754, -187.0858) (-2.8661, -187.2012) (-2.7749, -187.4018) knots 0 0 0 1 2 2 2
  spline S189 degree 2 poles (-2.7749, -187.4018) (-2.5015, -187.9912) (-1.7845, -187.9912) knots 0 0 0 1 1 1
  line L125 (-1.7845, -187.9912) -> (1.8614, -187.9912)
  line L126 (-0.2532, -193.8366) -> (0.6643, -193.1865)
  line L127 (0.6643, -193.1865) -> (2.0862, -193.1865)
  spline S190 degree 2 poles (2.0862, -193.1865) (2.5176, -193.1865) (2.9734, -192.8827) (3.1374, -192.5059) knots 0 0 0 1 2 2 2
  spline S191 degree 2 poles (3.1374, -192.5059) (3.186, -192.3722) (3.3076, -192.275) (3.3987, -192.275) knots 0 0 0 1 2 2 2
  spline S192 degree 2 poles (3.3987, -192.275) (3.5385, -192.275) (3.6661, -192.4938) (3.6661, -192.7307) knots 0 0 0 1 2 2 2
  line L128 (3.6661, -192.7307) -> (3.6661, -194.2681)
  spline S193 degree 2 poles (3.6661, -194.2681) (3.6661, -194.584) (3.581, -194.6813) knots 0 0 0 1 1 1
  spline S194 degree 2 poles (3.581, -194.6813) (3.502, -194.7846) (3.3866, -194.7846) knots 0 0 0 1 1 1
  spline S195 degree 2 poles (3.3866, -194.7846) (3.2833, -194.7846) (3.1739, -194.6691) (3.0827, -194.4443) knots 0 0 0 1 2 2 2
  spline S196 degree 2 poles (3.0827, -194.4443) (2.943, -194.1222) (2.6574, -193.9521) knots 0 0 0 1 1 1
  spline S197 degree 2 poles (2.6574, -193.9521) (2.4447, -193.8366) (2.0862, -193.8366) knots 0 0 0 1 1 1
  line L129 (2.0862, -193.8366) -> (-0.2532, -193.8366)
  line L130 (3.6661, -198.8983) -> (-3.3339, -198.8983)
  line L131 (-3.3339, -198.8983) -> (-3.3339, -196.1639)
  line L132 (-3.3339, -196.1639) -> (-3.3339, -196.0059)
  spline S198 degree 2 poles (-3.3339, -196.0059) (-3.3339, -195.7811) (-3.1942, -195.5441) (-3.0666, -195.5441) knots 0 0 0 1 2 2 2
  spline S199 degree 2 poles (-3.0666, -195.5441) (-2.86, -195.5441) (-2.7931, -195.7872) knots 0 0 0 1 1 1
  spline S200 degree 2 poles (-2.7931, -195.7872) (-2.7324, -195.9938) (-2.7081, -196.0606) (-2.6595, -196.0971) knots 0 0 0 1 2 2 2
  spline S201 degree 2 poles (-2.6595, -196.0971) (-2.5805, -196.17) (-2.3982, -196.17) knots 0 0 0 1 1 1
  line L133 (-2.3982, -196.17) -> (2.7303, -196.17)
  spline S202 degree 2 poles (2.7303, -196.17) (2.9126, -196.17) (2.9916, -196.0971) knots 0 0 0 1 1 1
  spline S203 degree 2 poles (2.9916, -196.0971) (3.0402, -196.0606) (3.0645, -195.9938) (3.1192, -195.7872) knots 0 0 0 1 2 2 2
  spline S204 degree 2 poles (3.1192, -195.7872) (3.186, -195.5441) (3.3987, -195.5441) knots 0 0 0 1 1 1
  spline S205 degree 2 poles (3.3987, -195.5441) (3.5263, -195.5441) (3.6661, -195.7811) (3.6661, -196.0059) knots 0 0 0 1 2 2 2
  line L134 (3.6661, -196.0059) -> (3.6661, -196.1639)
  line L135 (3.6661, -196.1639) -> (3.6661, -198.8983)
  line L136 (-3.3339, -199.4573) -> (-2.781, -199.4573)
  spline S206 degree 2 poles (-2.781, -199.4573) (-2.7324, -199.8584) (-2.544, -200.3809) (-2.3556, -200.6422) knots 0 0 0 1 2 2 2
  spline S207 degree 2 poles (-2.3556, -200.6422) (-2.1673, -200.9096) (-1.7602, -201.2195) (-1.4259, -201.3653) knots 0 0 0 1 2 2 2
  spline S208 degree 2 poles (-1.4259, -201.3653) (-1.2619, -201.4321) (-1.1464, -201.578) (-1.1464, -201.7056) knots 0 0 0 1 2 2 2
  spline S209 degree 2 poles (-1.1464, -201.7056) (-1.1464, -201.8818) (-1.3166, -202.0155) (-1.5232, -202.0155) knots 0 0 0 1 2 2 2
  line L137 (-1.5232, -202.0155) -> (-3.3339, -202.0155)
  line L138 (-3.3339, -202.0155) -> (-3.3339, -199.4573)
  line L139 (3.6661, -199.4512) -> (3.6661, -201.9304)
  line L140 (3.6661, -201.9304) -> (1.8492, -201.9304)
  spline S210 degree 2 poles (1.8492, -201.9304) (1.6912, -201.9304) (1.5515, -201.7846) (1.5515, -201.6205) knots 0 0 0 1 2 2 2
  spline S211 degree 2 poles (1.5515, -201.6205) (1.5515, -201.4868) (1.6426, -201.3653) (1.7885, -201.3106) knots 0 0 0 1 2 2 2
  spline S212 degree 2 poles (1.7885, -201.3106) (2.3779, -201.0736) (3.0037, -200.1682) (3.0645, -199.4512) knots 0 0 0 1 2 2 2
  line L141 (3.0645, -199.4512) -> (3.6661, -199.4512)
  line L142 (-0.0709, -199.4209) -> (0.5246, -199.4209)
  spline S213 degree 2 poles (0.5246, -199.4209) (0.6704, -199.7794) (1.0107, -200.1196) (1.2902, -200.2047) knots 0 0 0 1 2 2 2
  spline S214 degree 2 poles (1.2902, -200.2047) (1.4846, -200.2533) (1.6366, -200.4113) (1.6366, -200.5571) knots 0 0 0 1 2 2 2
  spline S215 degree 2 poles (1.6366, -200.5571) (1.6366, -200.7577) (1.5089, -200.8306) knots 0 0 0 1 1 1
  spline S216 degree 2 poles (1.5089, -200.8306) (1.4421, -200.8731) (1.2051, -200.8731) knots 0 0 0 1 1 1
  line L143 (1.2051, -200.8731) -> (-0.7515, -200.8731)
  spline S217 degree 2 poles (-0.7515, -200.8731) (-0.9945, -200.8731) (-1.1768, -200.7455) (-1.1768, -200.5693) knots 0 0 0 1 2 2 2
  spline S218 degree 2 poles (-1.1768, -200.5693) (-1.1768, -200.4295) (-1.031, -200.2715) (-0.8608, -200.2229) knots 0 0 0 1 2 2 2
  spline S219 degree 2 poles (-0.8608, -200.2229) (-0.5084, -200.1136) (-0.1317, -199.7307) (-0.0709, -199.4209) knots 0 0 0 1 2 2 2
  line L144 (3.6661, -206.2932) -> (-2.3617, -206.2932)
  spline S220 degree 2 poles (-2.3617, -206.2932) (-2.5622, -206.2932) (-2.6473, -206.3844) knots 0 0 0 1 1 1
  spline S221 degree 2 poles (-2.6473, -206.3844) (-2.6959, -206.433) (-2.7263, -206.5241) (-2.7749, -206.7611) knots 0 0 0 1 2 2 2
  spline S222 degree 2 poles (-2.7749, -206.7611) (-2.8296, -207.0589) (-3.0544, -207.0589) knots 0 0 0 1 1 1
  spline S223 degree 2 poles (-3.0544, -207.0589) (-3.1881, -207.0589) (-3.2732, -206.9009) knots 0 0 0 1 1 1
  spline S224 degree 2 poles (-3.2732, -206.9009) (-3.3339, -206.7794) (-3.3339, -206.512) knots 0 0 0 1 1 1
  line L145 (-3.3339, -206.512) -> (-3.3339, -206.2993)
  line L146 (-3.3339, -206.2993) -> (-3.3339, -203.5589)
  line L147 (-3.3339, -203.5589) -> (-3.3339, -203.4009)
  spline S225 degree 2 poles (-3.3339, -203.4009) (-3.3339, -203.1761) (-3.1942, -202.9391) (-3.0666, -202.9391) knots 0 0 0 1 2 2 2
  spline S226 degree 2 poles (-3.0666, -202.9391) (-2.86, -202.9391) (-2.7931, -203.1821) knots 0 0 0 1 1 1
  spline S227 degree 2 poles (-2.7931, -203.1821) (-2.7324, -203.3887) (-2.7081, -203.4556) (-2.6595, -203.492) knots 0 0 0 1 2 2 2
  spline S228 degree 2 poles (-2.6595, -203.492) (-2.5805, -203.5649) (-2.3982, -203.5649) knots 0 0 0 1 1 1
  line L148 (-2.3982, -203.5649) -> (2.7303, -203.5649)
  spline S229 degree 2 poles (2.7303, -203.5649) (2.9126, -203.5649) (2.9916, -203.492) knots 0 0 0 1 1 1
  spline S230 degree 2 poles (2.9916, -203.492) (3.0402, -203.4556) (3.0645, -203.3887) (3.1192, -203.1821) knots 0 0 0 1 2 2 2
  spline S231 degree 2 poles (3.1192, -203.1821) (3.186, -202.9391) (3.3987, -202.9391) knots 0 0 0 1 1 1
  spline S232 degree 2 poles (3.3987, -202.9391) (3.5263, -202.9391) (3.6661, -203.1761) (3.6661, -203.4009) knots 0 0 0 1 2 2 2
  line L149 (3.6661, -203.4009) -> (3.6661, -203.5589)
  line L150 (3.6661, -203.5589) -> (3.6661, -206.2932)
  spline S233 degree 2 poles (0.0931, -208.183) (0.0263, -208.7481) (-0.1499, -209.3618) (-0.3018, -209.6049) knots 0 0 0 1 2 2 2
  spline S234 degree 2 poles (-0.3018, -209.6049) (-0.4598, -209.8601) (-0.8973, -210.1396) (-1.1464, -210.1396) knots 0 0 0 1 2 2 2
  line L151 (-1.1464, -210.1396) -> (-2.2037, -210.1396)
  spline S235 degree 2 poles (-2.2037, -210.1396) (-2.3739, -210.1396) (-2.3739, -210.2672) knots 0 0 0 1 1 1
  spline S236 degree 2 poles (-2.3739, -210.2672) (-2.3739, -210.3158) (-2.3253, -210.3887) (-2.2584, -210.4495) knots 0 0 0 1 2 2 2
  spline S237 degree 2 poles (-2.2584, -210.4495) (-2.0822, -210.6014) (-2.0822, -210.7594) knots 0 0 0 1 1 1
  spline S238 degree 2 poles (-2.0822, -210.7594) (-2.0822, -210.8688) (-2.2645, -211.0754) (-2.3617, -211.0754) knots 0 0 0 1 2 2 2
  spline S239 degree 2 poles (-2.3617, -211.0754) (-2.5197, -211.0754) (-2.9754, -210.7108) (-3.1577, -210.4434) knots 0 0 0 1 2 2 2
  spline S240 degree 2 poles (-3.1577, -210.4434) (-3.3218, -210.1882) (-3.4737, -209.5988) (-3.4737, -209.1978) knots 0 0 0 1 2 2 2
  spline S241 degree 2 poles (-3.4737, -209.1978) (-3.4737, -208.3896) (-2.6959, -207.4781) (-2.0093, -207.4781) knots 0 0 0 1 2 2 2
  line L152 (-2.0093, -207.4781) -> (-1.1464, -207.4781)
  spline S242 degree 2 poles (-1.1464, -207.4781) (-0.8608, -207.4781) (-0.8122, -207.4721) knots 0 0 0 1 1 1
  spline S243 degree 2 poles (-0.8122, -207.4721) (-0.6056, -207.4417) (-0.4598, -207.3019) knots 0 0 0 1 1 1
  spline S244 degree 2 poles (-0.4598, -207.3019) (-0.2775, -207.1196) (-0.2471, -206.7915) knots 0 0 0 1 1 1
  line L153 (-0.2471, -206.7915) -> (0.2997, -206.7915)
  spline S245 degree 2 poles (0.2997, -206.7915) (0.3423, -207.1196) (0.4456, -207.2655) knots 0 0 0 1 1 1
  spline S246 degree 2 poles (0.4456, -207.2655) (0.5367, -207.387) (0.7737, -207.4781) (1.0046, -207.4781) knots 0 0 0 1 2 2 2
  line L154 (1.0046, -207.4781) -> (2.3657, -207.4781)
  spline S247 degree 2 poles (2.3657, -207.4781) (2.6878, -207.4781) (3.0037, -207.1743) (3.0949, -206.7854) knots 0 0 0 1 2 2 2
  line L155 (3.0949, -206.7854) -> (3.6661, -206.7854)
  line L156 (3.6661, -206.7854) -> (3.6661, -206.9434)
  spline S248 degree 2 poles (3.6661, -206.9434) (3.6661, -207.624) (3.6235, -208.104) knots 0 0 0 1 1 1
  spline S249 degree 2 poles (3.6235, -208.104) (3.5688, -208.8149) (3.2346, -209.374) knots 0 0 0 1 1 1
  spline S250 degree 2 poles (3.2346, -209.374) (2.7607, -210.1821) (1.8735, -210.1821) knots 0 0 0 1 1 1
  spline S251 degree 2 poles (1.8735, -210.1821) (1.1504, -210.1821) (0.6886, -209.6413) knots 0 0 0 1 1 1
  spline S252 degree 2 poles (0.6886, -209.6413) (0.4942, -209.4165) (0.2511, -208.8028) (0.0931, -208.183) knots 0 0 0 1 2 2 2
  point P0 (0, 0)
  constraints: 2 other
extrude "Extrusion3" cut sketch "Skizze8" against normal blind 10
equation "\"d125\" = Stärke"
equation "\"d6\" = Stärke"
equation "\"d7\" = BreiteBiegungsfreistellung"
equation "\"d8\" = TiefeBiegungsfreistellung"
equation "\"d9\" = MinimalRest"
equation "\"d10\" = Übergangsradius"
equation "\"d13\" = Biegeradius"
equation "\"d14\" = GrößeEckenfreistellung"
equation "\"d15\" = Abstandsgröße"
equation "\"d16\" = JacobiRadiusGröße"
equation "\"d17\" = BreiteBiegungsfreistellung"
equation "\"d18\" = TiefeBiegungsfreistellung"
equation "\"d19\" = MinimalRest"
equation "\"d20\" = Übergangsradius"
equation "\"d23\" = Biegeradius"
equation "\"d24\" = GrößeEckenfreistellung"
equation "\"d25\" = Abstandsgröße"
equation "\"d26\" = JacobiRadiusGröße"
equation "\"Biegeradius\" = Stärke"
equation "\"BreiteBiegungsfreistellung\" = Stärke"
equation "\"TiefeBiegungsfreistellung\" = 0.5 * Stärke"
equation "\"GrößeEckenfreistellung\" = 4 * Stärke"
equation "\"MinimalRest\" = 2 * Stärke"
equation "\"Übergangsradius\" = Biegeradius"
equation "\"JacobiRadiusGröße\" = Biegeradius"
equation "\"Abstandsgröße\" = Stärke"
equation "\"Stärke\" = 2"
